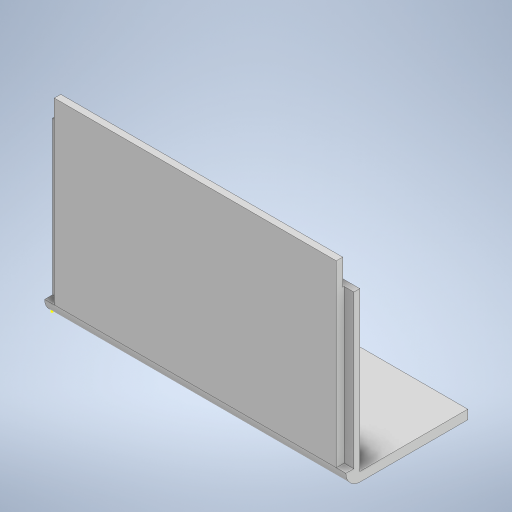
# Autodesk Inventor part: Lid Cover
Saved by Autodesk Inventor 2023 (Build 270158000, 158)
## iProperties
Created: 2024-03-25
Part Number: Lid Cover
Material: Generic
Document SubType Name: Modeling
Designer: Pobe Tran
Density: 1 g/cm^3
Appearance: Default
Author: Pobe Tran
Autodesk Inventor part; units mm, degrees
ref_plane "YZ Plane" through (0, 0, 0) normal (1, 0, 0) x (0, 1, 0)
ref_plane "XZ Plane" through (0, 0, 0) normal (0, 1, 0) x (-1, 0, 0)
ref_plane "XY Plane" through (0, 0, 0) normal (0, 0, 1) x (1, 0, 0)
sketch "Sketch1" plane through (0, 0, 0) normal (1, 0, 0) x (0, 1, 0)
  arc A0 (3.175, 26.5) -> (0, 23.325) centre (3.175, 23.325) ccw
  line L0 (36.4678, 26.5) -> (3.175, 26.5)
  line L1 (36.4678, 26.5) -> (36.4678, 23.5)
  line L2 (2, 23.5) -> (36.4678, 23.5)
  line L3 (2, 0) -> (2, 23.5)
  line L4 (0, 0) -> (2, 0)
  line L5 (0, 23.325) -> (0, 0)
  point P0 (0, 0)
  constraints: 12 end point, 2 point on circle, 1 centre point
extrude "Extrusion1" add sketch "Sketch1" along normal blind 65.626
sketch "Sketch2" plane through (0, 3.175, 26.5) normal (0, 0, 1) x (1, 0, 0)
  line L0 (0, 33.2928) -> (65.626, 33.2928) projected
  line L1 (7.465, 33.2928) -> (58.161, 33.2928)
  line L2 (58.161, 33.2928) -> (58.161, 39.4648)
  line L3 (58.161, 39.4648) -> (7.465, 39.4648)
  line L4 (7.465, 39.4648) -> (7.465, 33.2928)
  point P0 (0, -3.175)
  point P1 (32.813, 39.4648)
  point P2 (32.813, 33.2928)
  dimension "d2" = 50.696
  dimension "d3" = 6.172
  constraints: 8 end point, 2 midpoint, 2 parallel, 1 horizontal, 1 perpendicular, 1 point on line, 1 vertical alignment
  measures "d2" distance of L3.end L2.end
  measures "d3" distance of L3.end L1.start
extrude "Extrusion2" add sketch "Sketch2" against normal blind 1.7
sketch "Sketch3" plane through (0, 36.4678, 26.5) normal (0, 1, 0) x (1, 0, 0)
  line L0 (58.161, 0) -> (65.626, 0) projected
  line L1 (65.626, 0) -> (63.626, 0)
  line L2 (63.626, 0) -> (63.626, 1.7)
  line L3 (63.626, 1.7) -> (65.626, 1.7)
  line L4 (65.626, 1.7) -> (65.626, 0)
  line L5 (0, 0) -> (7.465, 0) projected
  line L6 (0, 0) -> (2, 0)
  line L7 (2, 0) -> (2, 1.7)
  line L8 (2, 1.7) -> (0, 1.7)
  line L9 (0, 1.7) -> (0, 0)
  point P0 (0, 26.5)
  point P1 (63.626, 0)
  dimension "d6" = 2
  dimension "d7" = 1.7
  dimension "d8" = 2
  dimension "d9" = 1.7
  constraints: 16 end point, 4 parallel, 2 horizontal, 2 perpendicular
  measures "d6" distance of L2.end L3.end
  measures "d7" distance of L1.end L2.end
  measures "d8" distance of L8.end L7.end
  measures "d9" distance of L7.end L6.end
extrude "Extrusion3" cut sketch "Sketch3" against normal up to surface (33.2928 mm away)
sketch "Sketch4" plane through (0, 36.4678, 23.5) normal (0, 1, 0) x (1, 0, 0)
  line L0 (2, -1.3) -> (2, -3) projected
  line L1 (63.626, -3) -> (2, -3)
  line L2 (2, -3) -> (2, -1.3)
  line L3 (2, -1.3) -> (63.626, -1.3)
  line L4 (63.626, -1.3) -> (63.626, -3)
  point P0 (0, 23.5)
  constraints: 8 end point, 2 parallel, 1 horizontal, 1 perpendicular
extrude "Extrusion4" add sketch "Sketch4" along normal up to surface (6.172 mm away)
sketch "Sketch5" plane through (0, 3.175, 24.8) normal (0, 0, -1) x (-1, 0, 0)
  point P0 (0, -3.175)
move faces "Move1" translate (0, 0, 0.3) faces at (43.084, 40.5825, 24.8)
move faces "Move2" translate (0.2, 0, 0) faces at (2, 27.4275, 25.9333)
move faces "Move3" translate (-0.1, 0, 0) faces at (63.626, 27.4275, 26.0333)
move faces "Move4" translate (0, -0.5, 0) faces at (22.642, 42.6398, 26.0333)
move faces "Move5" translate (0.1, 0, 0) faces at (0, 1.3333, 15.6083)
body "Solid1"
